Autodesk Fusion 360 part; units mm, degrees
note: some values were not read from the file. Chosen so that the rebuilt part matches the saved one: which bodies a step acts on.
(part 4 of 4)
  line L261 (1478.3146, -937.046) -> (1507.8943, -937.046)
  arc A56 (1474.0012, -558.7326) -> (1478.3146, -563.046) centre (1476.1579, -560.8893) ccw
  arc A57 (1217.2116, -740.7254) -> (1215.6328, -746.6175) centre (1216.4222, -743.6714) ccw
  arc A58 (1231.3944, -737.5175) -> (1225.5023, -735.9387) centre (1228.4484, -736.7281) ccw
  arc A59 (1270.6023, -814.0542) -> (1272.1811, -808.1621) centre (1271.3917, -811.1081) ccw
  arc A60 (1256.4194, -817.2621) -> (1262.3116, -818.8409) centre (1259.3655, -818.0515) ccw
  arc A61 (1001.2498, -651.7398) -> (996.9364, -656.0531) centre (999.0931, -653.8965) ccw
  arc A62 (1087.1364, -656.0531) -> (1082.823, -651.7398) centre (1084.9797, -653.8965) ccw
  arc A63 (1082.823, -669.9398) -> (1087.1364, -665.6264) centre (1084.9797, -667.7831) ccw
  arc A64 (996.9364, -665.6264) -> (1001.2498, -669.9398) centre (999.0931, -667.7831) ccw
  arc A65 (1262.3116, -502.8387) -> (1256.4194, -504.4175) centre (1259.3655, -503.6281) ccw
  arc A66 (1272.1811, -513.5175) -> (1270.6023, -507.6254) centre (1271.3917, -510.5714) ccw
  arc A67 (1225.5023, -585.7409) -> (1231.3944, -584.1621) centre (1228.4484, -584.9515) ccw
  arc A68 (1215.6328, -575.0621) -> (1217.2116, -580.9542) centre (1216.4222, -578.0081) ccw
  arc A69 (1589.3944, -164.7325) -> (1593.7078, -169.0459) centre (1591.5511, -166.8892) ccw
  arc A70 (1535.0811, -169.0459) -> (1539.3944, -164.7325) centre (1537.2378, -166.8892) ccw
  arc A71 (1539.3944, -547.3592) -> (1535.0811, -543.0459) centre (1537.2378, -545.2026) ccw
  arc A72 (1593.7078, -543.0459) -> (1589.3944, -547.3592) centre (1591.5511, -545.2026) ccw
  line L262 (1623.2875, -169.0459) -> (1593.7078, -169.0459)
  arc A73 (1451.6083, -128.7325) -> (1455.9216, -133.0458) centre (1453.765, -130.8892) ccw
  arc A74 (1397.2949, -133.0458) -> (1401.6083, -128.7325) centre (1399.4516, -130.8892) ccw
  arc A75 (1401.6083, -511.3592) -> (1397.2949, -507.0458) centre (1399.4516, -509.2025) ccw
  arc A76 (1455.9216, -507.0458) -> (1451.6083, -511.3592) centre (1453.765, -509.2025) ccw
  line L263 (1485.5013, -133.0458) -> (1455.9216, -133.0458)
  arc A77 (1161.2828, -393.1924) -> (1155.3907, -391.6136) centre (1158.3367, -392.403) ccw
  arc A78 (1180.4907, -435.0881) -> (1182.0695, -429.196) centre (1181.2801, -432.142) ccw
  arc A79 (1166.3078, -438.296) -> (1172.1999, -439.8748) centre (1169.2539, -439.0854) ccw
  arc A80 (1147.0999, -396.4003) -> (1145.5211, -402.2924) centre (1146.3105, -399.3464) ccw
  arc A81 (1172.1999, -280.6079) -> (1166.3078, -282.1867) centre (1169.2539, -281.3973) ccw
  arc A82 (1182.0695, -291.2867) -> (1180.4907, -285.3945) centre (1181.2801, -288.3406) ccw
  arc A83 (1155.3907, -328.869) -> (1161.2828, -327.2902) centre (1158.3367, -328.0796) ccw
  arc A84 (1145.5211, -318.1902) -> (1147.0999, -324.0823) centre (1146.3105, -321.1363) ccw
  arc A85 (1046.8748, -351.1413) -> (1042.5615, -355.4547) centre (1044.7182, -353.298) ccw
  arc A86 (1092.7615, -355.4547) -> (1088.4481, -351.1413) centre (1090.6048, -353.298) ccw
  arc A87 (1088.4481, -369.3413) -> (1092.7615, -365.028) centre (1090.6048, -367.1846) ccw
  arc A88 (1042.5615, -365.028) -> (1046.8748, -369.3413) centre (1044.7182, -367.1846) ccw
  arc A89 (814.3842, -589.1133) -> (810.0709, -584.7999) centre (812.2276, -586.9566) ccw
  arc A90 (908.6976, -584.7999) -> (904.3842, -589.1133) centre (906.5409, -586.9566) ccw
  arc A91 (904.3842, -170.4866) -> (908.6976, -174.7999) centre (906.5409, -172.6433) ccw
  arc A92 (810.0709, -174.7999) -> (814.3842, -170.4866) centre (812.2276, -172.6433) ccw
  line L264 (810.0709, -174.7999) -> (730, -174.7999)
  arc A93 (814.3842, -123.1133) -> (810.0709, -118.7999) centre (812.2276, -120.9566) ccw
  arc A94 (908.6976, -118.7999) -> (904.3842, -123.1133) centre (906.5409, -120.9566) ccw
  arc A95 (904.3842, 295.5134) -> (908.6976, 291.2001) centre (906.5409, 293.3567) ccw
  arc A96 (810.0709, 291.2001) -> (814.3842, 295.5134) centre (812.2276, 293.3567) ccw
  line L265 (730, -118.7999) -> (810.0709, -118.7999)
  arc A97 (1190.1758, -28.7607) -> (1184.2837, -27.1819) centre (1187.2298, -27.9713) ccw
  arc A98 (1209.3837, -70.6564) -> (1210.9625, -64.7642) centre (1210.1731, -67.7103) ccw
  arc A99 (1195.2008, -73.8642) -> (1201.093, -75.443) centre (1198.1469, -74.6536) ccw
  arc A100 (1175.993, -31.9685) -> (1174.4142, -37.8607) centre (1175.2036, -34.9146) ccw
  arc A101 (1268.0355, -97.7153) -> (1263.7221, -102.0287) centre (1265.8788, -99.872) ccw
  arc A102 (1313.9221, -102.0287) -> (1309.6088, -97.7153) centre (1311.7655, -99.872) ccw
  arc A103 (1309.6088, -115.9153) -> (1313.9221, -111.602) centre (1311.7655, -113.7587) ccw
  arc A104 (1263.7221, -111.602) -> (1268.0355, -115.9153) centre (1265.8788, -113.7587) ccw
  arc A105 (1201.093, -138.1877) -> (1195.2008, -139.7665) centre (1198.1469, -138.9771) ccw
  arc A106 (1210.9625, -148.8665) -> (1209.3837, -142.9743) centre (1210.1731, -145.9204) ccw
  arc A107 (1184.2837, -186.4488) -> (1190.1758, -184.87) centre (1187.2298, -185.6594) ccw
  arc A108 (1174.4142, -175.77) -> (1175.993, -181.6621) centre (1175.2036, -178.7161) ccw
  arc A109 (1451.6084, 301.2675) -> (1455.9217, 296.9541) centre (1453.765, 299.1108) ccw
  arc A110 (1397.295, 296.9541) -> (1401.6084, 301.2675) centre (1399.4517, 299.1108) ccw
  arc A111 (1401.6084, -81.3592) -> (1397.295, -77.0459) centre (1399.4517, -79.2026) ccw
  arc A112 (1455.9217, -77.0459) -> (1451.6084, -81.3592) centre (1453.765, -79.2026) ccw
  line L266 (1485.5014, 296.9541) -> (1455.9217, 296.9541)
  arc A113 (1589.3944, 265.2675) -> (1593.7078, 260.9541) centre (1591.5511, 263.1108) ccw
  arc A114 (1535.0811, 260.9541) -> (1539.3944, 265.2675) centre (1537.2377, 263.1108) ccw
  arc A115 (1539.3944, -117.3592) -> (1535.0811, -113.0459) centre (1537.2377, -115.2026) ccw
  arc A116 (1593.7078, -113.0459) -> (1589.3944, -117.3592) centre (1591.5511, -115.2026) ccw
  line L267 (1623.2875, 260.9541) -> (1593.7078, 260.9541)
  arc A117 (1589.3945, 695.2675) -> (1593.7079, 690.9541) centre (1591.5512, 693.1108) ccw
  arc A118 (1535.0812, 690.9541) -> (1539.3945, 695.2675) centre (1537.2379, 693.1108) ccw
  arc A119 (1539.3945, 312.6408) -> (1535.0812, 316.9541) centre (1537.2379, 314.7974) ccw
  arc A120 (1593.7079, 316.9541) -> (1589.3945, 312.6408) centre (1591.5512, 314.7974) ccw
  line L268 (1623.2876, 690.9541) -> (1593.7079, 690.9541)
  arc A121 (1451.6084, 731.2675) -> (1455.9217, 726.9541) centre (1453.7651, 729.1108) ccw
  arc A122 (1397.295, 726.9541) -> (1401.6084, 731.2675) centre (1399.4517, 729.1108) ccw
  arc A123 (1401.6084, 348.6408) -> (1397.295, 352.9541) centre (1399.4517, 350.7974) ccw
  arc A124 (1455.9217, 352.9541) -> (1451.6084, 348.6408) centre (1453.7651, 350.7974) ccw
  line L269 (1485.5014, 726.9541) -> (1455.9217, 726.9541)
  arc A125 (1161.2829, 113.6596) -> (1155.3907, 115.2384) centre (1158.3368, 114.449) ccw
  arc A126 (1180.4907, 71.7639) -> (1182.0695, 77.6561) centre (1181.2801, 74.71) ccw
  arc A127 (1166.3078, 68.5561) -> (1172.2, 66.9773) centre (1169.2539, 67.7667) ccw
  arc A128 (1147.1, 110.4518) -> (1145.5212, 104.5596) centre (1146.3106, 107.5057) ccw
  arc A129 (1046.8749, 155.7107) -> (1042.5615, 151.3974) centre (1044.7182, 153.5541) ccw
  arc A130 (1092.7615, 151.3974) -> (1088.4482, 155.7107) centre (1090.6049, 153.5541) ccw
  arc A131 (1088.4482, 137.5107) -> (1092.7615, 141.8241) centre (1090.6049, 139.6674) ccw
  arc A132 (1042.5615, 141.8241) -> (1046.8749, 137.5107) centre (1044.7182, 139.6674) ccw
  arc A133 (1172.2, 226.2442) -> (1166.3078, 224.6654) centre (1169.2539, 225.4548) ccw
  arc A134 (1182.0695, 215.5654) -> (1180.4907, 221.4575) centre (1181.2801, 218.5115) ccw
  arc A135 (1155.3907, 177.9831) -> (1161.2829, 179.5619) centre (1158.3368, 178.7725) ccw
  arc A136 (1145.5212, 188.6619) -> (1147.1, 182.7697) centre (1146.3106, 185.7158) ccw
  arc A137 (1190.176, 478.0913) -> (1184.2838, 479.6701) centre (1187.2299, 478.8807) ccw
  arc A138 (1209.3838, 436.1957) -> (1210.9626, 442.0878) centre (1210.1732, 439.1417) ccw
  arc A139 (1195.2009, 432.9878) -> (1201.0931, 431.409) centre (1198.147, 432.1984) ccw
  arc A140 (1175.9931, 474.8835) -> (1174.4143, 468.9913) centre (1175.2037, 471.9374) ccw
  arc A141 (1201.0931, 368.6644) -> (1195.2009, 367.0856) centre (1198.147, 367.875) ccw
  arc A142 (1210.9626, 357.9856) -> (1209.3838, 363.8777) centre (1210.1732, 360.9316) ccw
  arc A143 (1184.2838, 320.4032) -> (1190.176, 321.982) centre (1187.2299, 321.1926) ccw
  arc A144 (1174.4143, 331.082) -> (1175.9931, 325.1899) centre (1175.2037, 328.136) ccw
  arc A145 (1268.0356, 409.1367) -> (1263.7223, 404.8233) centre (1265.8789, 406.98) ccw
  arc A146 (1313.9223, 404.8233) -> (1309.6089, 409.1367) centre (1311.7656, 406.98) ccw
  arc A147 (1309.6089, 390.9367) -> (1313.9223, 395.25) centre (1311.7656, 393.0934) ccw
  arc A148 (1263.7223, 395.25) -> (1268.0356, 390.9367) centre (1265.8789, 393.0934) ccw
  arc A149 (1092.7616, 658.25) -> (1088.4482, 662.5633) centre (1090.6049, 660.4066) ccw
  arc A150 (1088.4482, 644.3633) -> (1092.7616, 648.6767) centre (1090.6049, 646.52) ccw
  arc A151 (1042.5616, 648.6767) -> (1046.875, 644.3633) centre (1044.7183, 646.52) ccw
  arc A152 (1046.875, 662.5633) -> (1042.5616, 658.25) centre (1044.7183, 660.4066) ccw
  arc A153 (1161.2829, 620.5122) -> (1155.3908, 622.091) centre (1158.3369, 621.3016) ccw
  arc A154 (1180.4908, 578.6165) -> (1182.0696, 584.5087) centre (1181.2802, 581.5626) ccw
  arc A155 (1166.3079, 575.4087) -> (1172.2001, 573.8299) centre (1169.254, 574.6193) ccw
  arc A156 (1147.1001, 617.3043) -> (1145.5213, 611.4122) centre (1146.3107, 614.3583) ccw
  arc A157 (1172.2001, 733.0968) -> (1166.3079, 731.518) centre (1169.254, 732.3074) ccw
  arc A158 (1182.0696, 722.418) -> (1180.4908, 728.3101) centre (1181.2802, 725.364) ccw
  arc A159 (1155.3908, 684.8356) -> (1161.2829, 686.4144) centre (1158.3369, 685.625) ccw
  arc A160 (1145.5213, 695.5144) -> (1147.1001, 689.6223) centre (1146.3107, 692.5684) ccw
  arc A161 (814.3842, 342.8867) -> (810.0709, 347.2001) centre (812.2276, 345.0434) ccw
  arc A162 (908.6976, 347.2001) -> (904.3842, 342.8867) centre (906.5409, 345.0434) ccw
  arc A163 (904.3842, 761.5134) -> (908.6976, 757.2001) centre (906.5409, 759.3567) ccw
  arc A164 (810.0709, 757.2001) -> (814.3842, 761.5134) centre (812.2276, 759.3567) ccw
  line L270 (730, 347.2001) -> (810.0709, 347.2001)
  point P0 (700, -1519.2)
  point P1 (700, 919.2)
  dimension "d106" = 1220
  constraint horizontal L255
  constraint vertical L256
  constraint horizontal L257
  constraint vertical L258
  constraint coincident P0 L255.start
  constraint coincident P1 L257
  measures "d106" distance of P0 L255.end
component "sheet" placed x (1, 0, 0) y (0, 1, 0) z (0, 0, 1) at (0, 0, 0)
component "Table" placed x (1, 0, 0) y (0, 1, 0) z (0, 0, 1) at (0, 0, 0)
component "Chair 1" placed x (1, 0, 0) y (0, 1, 0) z (0, 0, 1) at (0, 0, 0)
component "Chair 2" placed x (1, 0, 0) y (0, 1, 0) z (0, 0, 1) at (0, 0, 0)
component "Chair 3" placed x (1, 0, 0) y (0, 1, 0) z (0, 0, 1) at (0, 0, 0)
component "Arrange1" placed x (1, 0, 0) y (0, 1, 0) z (0, 0, 1) at (0, 0, 0)
component "Component" placed x (1, 0, 0) y (0, 1, 0) z (0, 0, 1) at (0, 0, 0) in component "Table"
component "Component'''" placed x (1, 0, 0) y (0, 1, 0) z (0, 0, 1) at (0, 0, 0) in component "Table"
component "Component''" placed x (1, 0, 0) y (0, 1, 0) z (0, 0, 1) at (0, 0, 0) in component "Table"
component "Component'''''" placed x (1, 0, 0) y (0, 1, 0) z (0, 0, 1) at (0, 0, 0) in component "Table"
component "Component'" placed x (1, 0, 0) y (0, 1, 0) z (0, 0, 1) at (0, 0, 0) in component "Table"
component "Component'''''''''''" placed x (1, 0, 0) y (0, 1, 0) z (0, 0, 1) at (0, 0, 0) in component "Chair 1"
component "Component'''''''''''''" placed x (1, 0, 0) y (0, 1, 0) z (0, 0, 1) at (0, 0, 0) in component "Chair 1"
component "Component'''''''''''''''" placed x (1, 0, 0) y (0, 1, 0) z (0, 0, 1) at (0, 0, 0) in component "Chair 1"
component "Component'''''''''''''''''" placed x (1, 0, 0) y (0, 1, 0) z (0, 0, 1) at (0, 0, 0) in component "Chair 1"
component "Component'''''''''''''''''''" placed x (1, 0, 0) y (0, 1, 0) z (0, 0, 1) at (0, 0, 0) in component "Chair 1"
component "Component''''" placed x (1, 0, 0) y (0, 1, 0) z (0, 0, 1) at (0, 0, 0) in component "Chair 2"
component "Component''''''" placed x (1, 0, 0) y (0, 1, 0) z (0, 0, 1) at (0, 0, 0) in component "Chair 2"
component "Component'''''''''" placed x (1, 0, 0) y (0, 1, 0) z (0, 0, 1) at (0, 0, 0) in component "Chair 2"
component "Component''''''''" placed x (1, 0, 0) y (0, 1, 0) z (0, 0, 1) at (0, 0, 0) in component "Chair 2"
component "Component'''''''" placed x (1, 0, 0) y (0, 1, 0) z (0, 0, 1) at (0, 0, 0) in component "Chair 2"
component "Component''''''''''''''''''" placed x (1, 0, 0) y (0, 1, 0) z (0, 0, 1) at (0, 0, 0) in component "Chair 3"
component "Component''''''''''''''''" placed x (1, 0, 0) y (0, 1, 0) z (0, 0, 1) at (0, 0, 0) in component "Chair 3"
component "Component''''''''''''''" placed x (1, 0, 0) y (0, 1, 0) z (0, 0, 1) at (0, 0, 0) in component "Chair 3"
component "Component''''''''''''" placed x (1, 0, 0) y (0, 1, 0) z (0, 0, 1) at (0, 0, 0) in component "Chair 3"
component "Component''''''''''" placed x (1, 0, 0) y (0, 1, 0) z (0, 0, 1) at (0, 0, 0) in component "Chair 3"
component "Envelope1(Qty: 1)" placed x (0, 1, 0) y (0, 0, 1) z (1, 0, 0) at (19, 700, -1519.2) in component "Arrange1"
component "Component" placed x (0, 0, 1) y (0, -1, 0) z (1, 0, 0) at (293.9645, 474.5207, 20) in component "Envelope1(Qty: 1)"
component "Component'" placed x (0, 1, 0) y (0, 0, -1) z (-1, 0, 0) at (24.8039, 1344.4001, 29) in component "Envelope1(Qty: 1)"
component "Component''" placed x (0, -1, 0) y (0.866025, 0, -0.5) z (0.5, 0, 0.866025) at (24.8039, 1400.4001, 29) in component "Envelope1(Qty: 1)"
component "Component'''" placed x (0, -1, 0) y (0.866025, 0, 0.5) z (-0.5, 0, 0.866025) at (293.9646, 1866.4001, 29) in component "Envelope1(Qty: 1)"
component "Component'''''" placed x (0, 0, 1) y (0, -1, 0) z (1, 0, 0) at (476.6167, 858.3602, 448) in component "Envelope1(Qty: 1)"
component "Component'''''''''''" placed x (0, 0, 1) y (0.866025, -0.5, 0) z (0.5, 0.866025, 0) at (553.133, 459.4162, 56) in component "Envelope1(Qty: 1)"
component "Component'''''''''''''" placed x (0, 0, 1) y (-0.866025, 0.5, 0) z (-0.5, -0.866025, 0) at (563.5294, 929.8747, 448) in component "Envelope1(Qty: 1)"
component "Component'''''''''''''''" placed x (0, 1, 0) y (-0.866025, 0, -0.5) z (-0.5, 0, 0.866025) at (944.8691, 992.154, 258.084) in component "Envelope1(Qty: 1)"
component "Component'''''''''''''''''" placed x (0, -1, 0) y (0.866025, 0, 0.5) z (-0.5, 0, 0.866025) at (526.4156, 976.1542, 29.4183) in component "Envelope1(Qty: 1)"
component "Component'''''''''''''''''''" placed x (0, -1, 0) y (0, 0, -1) z (1, 0, 0) at (923.2008, 1406.1541, 257.6657) in component "Envelope1(Qty: 1)"
component "Component''''" placed x (0, 0, 1) y (0, -1, 0) z (1, 0, 0) at (563.733, 1437.2107, 56) in component "Envelope1(Qty: 1)"
component "Component''''''" placed x (0, 0, 1) y (0, 1, 0) z (-1, 0, 0) at (392.7507, 1640.9847, 448) in component "Envelope1(Qty: 1)"
component "Component'''''''" placed x (0, -1, 0) y (0, 0, -1) z (1, 0, 0) at (922.6799, 1836.1541, -199.6) in component "Envelope1(Qty: 1)"
component "Component''''''''" placed x (0, 1, 0) y (-0.866025, 0, -0.5) z (-0.5, 0, 0.866025) at (686.9118, 458, 29) in component "Envelope1(Qty: 1)"
component "Component'''''''''" placed x (0, -1, 0) y (0.866025, 0, 0.5) z (-0.5, 0, 0.866025) at (1082.8587, 442, 257.6) in component "Envelope1(Qty: 1)"
component "Component''''''''''" placed x (0, 0, 1) y (-0.866025, -0.5, 0) z (0.5, -0.866025, 0) at (393.2717, 2147.9024, 56) in component "Envelope1(Qty: 1)"
component "Component''''''''''''" placed x (0, 0, 1) y (0.866025, 0.5, 0) z (-0.5, 0.866025, 0) at (563.2121, 1943.9976, 448) in component "Envelope1(Qty: 1)"
component "Component''''''''''''''" placed x (0, -1, 0) y (0.866025, 0, 0.5) z (-0.5, 0, 0.866025) at (1059.945, 940.1541, -199.6657) in component "Envelope1(Qty: 1)"
component "Component''''''''''''''''" placed x (0, -1, 0) y (0, 0, -1) z (1, 0, 0) at (664.7226, 1370.1541, 29.484) in component "Envelope1(Qty: 1)"
component "Component''''''''''''''''''" placed x (0, -1, 0) y (0.866025, 0, -0.5) z (0.5, 0, 0.866025) at (668.0057, 1800.1541, -199.1817) in component "Envelope1(Qty: 1)"
equation "d1 = table_width"
equation "thickness = 18 mm"
equation "d3 = thickness / 2"
equation "d4 = -( thickness / 2 )"
equation "d5 = thickness / 2"
equation "d6 = thickness / 2"
equation "d7 = d6"
equation "d8 = d6"
equation "d9 = -thickness / 2"
equation "d10 = thickness / 2"
equation "d11 = thickness / 2"
equation "d12 = thickness"
equation "d14 = -table_height"
equation "d18 = -thickness"
equation "d19 = -thickness"
equation "d32 = thickness"
equation "d39 = thickness"
equation "clearance = 0.1 mm"
equation "d44 = -clearance"
equation "d52 = -clearance"
equation "table_width = 3 ft"
equation "table_height = 41 cm"
equation "dogbone = 6.1 mm"
equation "d525 = dogbone / 2"
equation "d533 = dogbone / 2"
equation "d541 = dogbone / 2"
equation "d549 = dogbone / 2"
equation "d557 = dogbone / 2"
equation "d565 = dogbone / 2"
equation "d573 = dogbone / 2"
equation "d581 = dogbone / 2"
equation "d589 = dogbone / 2"
equation "d597 = dogbone / 2"
equation "d605 = dogbone / 2"
equation "d613 = dogbone / 2"
equation "d621 = dogbone / 2"
equation "d629 = dogbone / 2"
equation "d637 = dogbone / 2"
equation "d645 = dogbone / 2"
equation "d653 = dogbone / 2"
equation "d661 = dogbone / 2"
equation "d669 = dogbone / 2"
equation "d677 = dogbone / 2"
equation "d685 = dogbone / 2"
equation "d693 = dogbone / 2"
equation "d701 = dogbone / 2"
equation "d709 = dogbone / 2"
equation "d717 = dogbone / 2"
equation "d725 = dogbone / 2"
equation "d733 = dogbone / 2"
equation "d741 = dogbone / 2"
equation "d749 = dogbone / 2"
equation "d757 = dogbone / 2"
equation "d765 = dogbone / 2"
equation "d773 = dogbone / 2"
equation "d781 = dogbone / 2"
equation "d789 = dogbone / 2"
equation "d797 = dogbone / 2"
equation "d805 = dogbone / 2"
equation "d813 = dogbone / 2"
equation "d821 = dogbone / 2"
equation "d829 = dogbone / 2"
equation "d837 = dogbone / 2"
equation "d845 = dogbone / 2"
equation "d853 = dogbone / 2"
equation "d861 = dogbone / 2"
equation "d869 = dogbone / 2"
equation "d877 = dogbone / 2"
equation "d885 = dogbone / 2"
equation "d893 = dogbone / 2"
equation "d901 = dogbone / 2"
equation "d909 = dogbone / 2"
equation "d917 = dogbone / 2"
equation "d925 = dogbone / 2"
equation "d933 = dogbone / 2"
equation "d941 = dogbone / 2"
equation "d949 = dogbone / 2"
equation "d957 = dogbone / 2"
equation "d965 = dogbone / 2"
equation "d973 = dogbone / 2"
equation "d981 = dogbone / 2"
equation "d989 = dogbone / 2"
equation "d997 = dogbone / 2"
equation "d1005 = dogbone / 2"
equation "d1013 = dogbone / 2"
equation "d1021 = dogbone / 2"
equation "d1029 = dogbone / 2"
equation "d1037 = dogbone / 2"
equation "d1045 = dogbone / 2"
equation "d1053 = dogbone / 2"
equation "d1061 = dogbone / 2"
equation "d1069 = dogbone / 2"
equation "d1077 = dogbone / 2"
equation "d1085 = dogbone / 2"
equation "d1093 = dogbone / 2"
equation "d1101 = dogbone / 2"
equation "d1109 = dogbone / 2"
equation "d1117 = dogbone / 2"
equation "d1125 = dogbone / 2"
equation "d1133 = dogbone / 2"
equation "d1141 = dogbone / 2"
equation "d1149 = dogbone / 2"
equation "d1157 = dogbone / 2"
equation "d1165 = dogbone / 2"
equation "d1173 = dogbone / 2"
equation "d1181 = dogbone / 2"
equation "d1189 = dogbone / 2"
equation "d1197 = dogbone / 2"
equation "d1205 = dogbone / 2"
equation "d1213 = dogbone / 2"
equation "d1221 = dogbone / 2"
equation "d1229 = dogbone / 2"
equation "d1237 = dogbone / 2"
equation "d1245 = dogbone / 2"
equation "d1253 = dogbone / 2"
equation "d1261 = dogbone / 2"
equation "d1269 = dogbone / 2"
equation "d1277 = dogbone / 2"
equation "d1285 = dogbone / 2"
equation "d1293 = dogbone / 2"
equation "d1301 = dogbone / 2"
equation "d1309 = dogbone / 2"
equation "d1317 = dogbone / 2"
equation "d1325 = dogbone / 2"
equation "d1333 = dogbone / 2"
equation "d1341 = dogbone / 2"
equation "d1349 = dogbone / 2"
equation "d1357 = dogbone / 2"
equation "d1365 = dogbone / 2"
equation "d1373 = dogbone / 2"
equation "d1381 = dogbone / 2"
equation "d1389 = dogbone / 2"
equation "d1397 = dogbone / 2"
equation "d1405 = dogbone / 2"
equation "d1413 = dogbone / 2"
equation "d1421 = dogbone / 2"
equation "d1429 = dogbone / 2"
equation "d1437 = dogbone / 2"
equation "d1445 = dogbone / 2"
equation "d1453 = dogbone / 2"
equation "d1461 = dogbone / 2"
equation "d1469 = dogbone / 2"
equation "d1477 = dogbone / 2"
equation "d1485 = dogbone / 2"
equation "d1493 = dogbone / 2"
equation "d1501 = dogbone / 2"
equation "d1509 = dogbone / 2"
equation "d1517 = dogbone / 2"
equation "d1525 = dogbone / 2"
equation "d1533 = dogbone / 2"
equation "d1541 = dogbone / 2"
equation "d1549 = dogbone / 2"
equation "d1557 = dogbone / 2"
equation "d1565 = dogbone / 2"
equation "d1573 = dogbone / 2"
equation "d1581 = dogbone / 2"
equation "d1589 = dogbone / 2"
equation "d1597 = dogbone / 2"
equation "d1605 = dogbone / 2"
equation "d1613 = dogbone / 2"
equation "d1621 = dogbone / 2"
equation "d1629 = dogbone / 2"
equation "d1637 = dogbone / 2"
equation "d1645 = dogbone / 2"
equation "d1653 = dogbone / 2"
equation "d1661 = dogbone / 2"
equation "d1669 = dogbone / 2"
